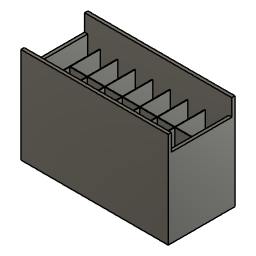
Box of WiFi (Autodesk Fusion 360 design; units mm, degrees)
Autodesk Fusion 360 part; units mm, degrees
sketch "Sketch1" plane through (0, 0, 0) normal (0, 1, 0) x (1, 0, 0)
  line L0 (0, 0) -> (139, 0)
  line L1 (139, 0) -> (139, -63)
  line L2 (139, -63) -> (0, -63)
  line L3 (0, -63) -> (0, 0)
  line L4 (0, 0) -> (139, 0)
  line L5 (139, 0) -> (139, -3)
  line L6 (139, -3) -> (0, -3)
  line L7 (0, -3) -> (0, 0)
  line L8 (0, -60) -> (139, -60)
  line L9 (139, -60) -> (139, -63)
  line L10 (139, -63) -> (0, -63)
  line L11 (0, -63) -> (0, -60)
  line L12 (136, -3) -> (139, -3)
  line L13 (139, -3) -> (139, -60)
  line L14 (139, -60) -> (136, -60)
  line L15 (136, -60) -> (136, -3)
  line L16 (0, -3) -> (3, -3)
  line L17 (3, -3) -> (3, -60)
  line L18 (3, -60) -> (0, -60)
  line L19 (0, -60) -> (0, -3)
  circle A0 centre (121.9, -46) radius 3.5
  line L20 (113.4, -3) -> (113.9, -3)
  line L21 (113.9, -3) -> (113.9, -60)
  line L22 (113.9, -60) -> (113.4, -60)
  line L23 (113.4, -60) -> (113.4, -3)
  circle A1 centre (121.9, -17) radius 3.5
  circle A2 centre (121.9, -46) radius 3.5
  line L24 (113.4, -3) -> (113.9, -3)
  line L25 (113.9, -60) -> (113.4, -60)
  line L26 (113.9, -3) -> (113.9, -60)
  circle A3 centre (121.9, -17) radius 3.5
  line L27 (113.4, -60) -> (113.4, -3)
  line L28 (96.9, -60) -> (96.9, -3)
  circle A4 centre (105.4, -46) radius 3.5
  line L29 (97.4, -60) -> (96.9, -60)
  line L30 (96.9, -3) -> (97.4, -3)
  line L31 (96.9, -3) -> (97.4, -3)
  circle A5 centre (105.4, -46) radius 3.5
  line L32 (97.4, -60) -> (96.9, -60)
  circle A6 centre (105.4, -17) radius 3.5
  line L33 (97.4, -3) -> (97.4, -60)
  line L34 (96.9, -60) -> (96.9, -3)
  circle A7 centre (105.4, -17) radius 3.5
  line L35 (97.4, -3) -> (97.4, -60)
  line L36 (80.9, -60) -> (80.4, -60)
  line L37 (80.4, -3) -> (80.9, -3)
  line L38 (80.4, -60) -> (80.4, -3)
  circle A8 centre (88.9, -17) radius 3.5
  line L39 (80.9, -3) -> (80.9, -60)
  circle A9 centre (88.9, -46) radius 3.5
  circle A10 centre (88.9, -17) radius 3.5
  line L40 (80.9, -3) -> (80.9, -60)
  line L41 (80.4, -60) -> (80.4, -3)
  line L42 (80.9, -60) -> (80.4, -60)
  line L43 (80.4, -3) -> (80.9, -3)
  circle A11 centre (88.9, -46) radius 3.5
  line L44 (63.9, -60) -> (63.9, -3)
  line L45 (63.9, -60) -> (63.9, -3)
  line L46 (64.4, -3) -> (64.4, -60)
  line L47 (64.4, -3) -> (64.4, -60)
  circle A12 centre (72.4, -46) radius 3.5
  circle A13 centre (72.4, -17) radius 3.5
  line L48 (63.9, -3) -> (64.4, -3)
  line L49 (63.9, -3) -> (64.4, -3)
  line L50 (64.4, -60) -> (63.9, -60)
  circle A14 centre (72.4, -46) radius 3.5
  circle A15 centre (72.4, -17) radius 3.5
  line L51 (64.4, -60) -> (63.9, -60)
  line L52 (47.4, -60) -> (47.4, -3)
  line L53 (47.9, -3) -> (47.9, -60)
  line L54 (47.4, -60) -> (47.4, -3)
  line L55 (47.4, -3) -> (47.9, -3)
  line L56 (47.4, -3) -> (47.9, -3)
  line L57 (47.9, -3) -> (47.9, -60)
  circle A16 centre (55.9, -17) radius 3.5
  circle A17 centre (55.9, -46) radius 3.5
  line L58 (47.9, -60) -> (47.4, -60)
  circle A18 centre (55.9, -46) radius 3.5
  circle A19 centre (55.9, -17) radius 3.5
  line L59 (47.9, -60) -> (47.4, -60)
  circle A20 centre (39.4, -17) radius 3.5
  line L60 (30.9, -3) -> (31.4, -3)
  circle A21 centre (39.4, -46) radius 3.5
  line L61 (30.9, -60) -> (30.9, -3)
  line L62 (30.9, -60) -> (30.9, -3)
  line L63 (31.4, -3) -> (31.4, -60)
  line L64 (30.9, -3) -> (31.4, -3)
  line L65 (31.4, -3) -> (31.4, -60)
  line L66 (31.4, -60) -> (30.9, -60)
  circle A22 centre (39.4, -17) radius 3.5
  circle A23 centre (39.4, -46) radius 3.5
  line L67 (31.4, -60) -> (30.9, -60)
  line L68 (14.9, -3) -> (14.9, -60)
  line L69 (14.4, -3) -> (14.9, -3)
  line L70 (14.4, -60) -> (14.4, -3)
  line L71 (14.9, -60) -> (14.4, -60)
  line L72 (14.9, -3) -> (14.9, -60)
  circle A24 centre (22.9, -46) radius 3.5
  line L73 (14.4, -60) -> (14.4, -3)
  circle A25 centre (22.9, -46) radius 3.5
  line L74 (14.4, -3) -> (14.9, -3)
  line L75 (14.9, -60) -> (14.4, -60)
  circle A26 centre (22.9, -17) radius 3.5
  circle A27 centre (22.9, -17) radius 3.5
  line L76 (130.4, -60) -> (129.9, -60)
  line L77 (129.9, -3) -> (130.4, -3)
  line L78 (130.4, -60) -> (129.9, -60)
  line L79 (129.9, -3) -> (130.4, -3)
  line L80 (129.9, -60) -> (129.9, -3)
  line L81 (130.4, -3) -> (130.4, -60)
  line L82 (129.9, -60) -> (129.9, -3)
  line L83 (130.4, -3) -> (130.4, -60)
  line L84 (14.9, -31.25) -> (129.9, -31.25)
  line L85 (129.9, -31.25) -> (129.9, -31.75)
  line L86 (129.9, -31.75) -> (14.9, -31.75)
  line L87 (14.9, -31.75) -> (14.9, -31.25)
  line L88 (120, -59) -> (124, -59)
  line L89 (124, -59) -> (124, -60)
  line L90 (124, -60) -> (120, -60)
  line L91 (120, -60) -> (120, -59)
  line L92 (103, -60) -> (107, -60)
  line L93 (107, -60) -> (107, -59)
  line L94 (107, -59) -> (103, -59)
  line L95 (103, -59) -> (103, -60)
  line L96 (21, -3) -> (25, -3)
  line L97 (25, -3) -> (25, -4)
  line L98 (25, -4) -> (21, -4)
  line L99 (21, -4) -> (21, -3)
  line L100 (37, -3) -> (41, -3)
  line L101 (41, -3) -> (41, -4)
  line L102 (41, -4) -> (37, -4)
  line L103 (37, -4) -> (37, -3)
  line L104 (21, -60) -> (25, -60)
  line L105 (25, -60) -> (25, -59)
  line L106 (25, -59) -> (21, -59)
  line L107 (21, -59) -> (21, -60)
  line L108 (37, -60) -> (41, -60)
  line L109 (41, -60) -> (41, -59)
  line L110 (41, -59) -> (37, -59)
  line L111 (37, -59) -> (37, -60)
  line L112 (103, -3) -> (107, -3)
  line L113 (107, -3) -> (107, -4)
  line L114 (107, -4) -> (103, -4)
  line L115 (103, -4) -> (103, -3)
  line L116 (120, -3) -> (124, -3)
  line L117 (124, -3) -> (124, -4)
  line L118 (124, -4) -> (120, -4)
  line L119 (120, -4) -> (120, -3)
  dimension "d1" = 139
  dimension "d2" = 63
  dimension "d3" = 139
  dimension "d4" = 3
  dimension "d5" = 139
  dimension "d6" = 3
  dimension "d7" = 7
  dimension "d8" = 14.1
  dimension "d9" = 14
  dimension "d10" = 0.5
  dimension "d11" = 8
  dimension "d12" = 7
  dimension "d13" = 14
  dimension "d14" = 7
  dimension "d15" = 0.5
  dimension "d16" = 8
  dimension "d17" = 7
  dimension "d18" = 7
  dimension "d19" = 0.5
  dimension "d20" = 8
  dimension "d21" = 7
  dimension "d22" = 7
  dimension "d23" = 0.5
  dimension "d24" = 8
  dimension "d25" = 7
  dimension "d26" = 7
  dimension "d27" = 0.5
  dimension "d28" = 8
  dimension "d29" = 7
  dimension "d30" = 7
  dimension "d31" = 0.5
  dimension "d32" = 8
  dimension "d33" = 7
  dimension "d34" = 7
  dimension "d35" = 0.5
  dimension "d36" = 8
  dimension "d37" = 7
  dimension "d38" = 7
  dimension "d39" = 0.5
  dimension "d40" = 8
  dimension "d41" = 7
  dimension "d42" = 7
  dimension "d43" = 0.5
  dimension "d44" = 8
  dimension "d45" = 7
  dimension "d46" = 7
  dimension "d47" = 0.5
  dimension "d48" = 8
  dimension "d49" = 7
  dimension "d50" = 7
  dimension "d51" = 0.5
  dimension "d52" = 8
  dimension "d53" = 7
  dimension "d54" = 7
  dimension "d55" = 0.5
  dimension "d56" = 8
  dimension "d57" = 7
  dimension "d58" = 7
  dimension "d59" = 0.5
  dimension "d60" = 8
  dimension "d61" = 7
  dimension "d62" = 7
  dimension "d63" = 0.5
  dimension "d64" = 8
  dimension "d65" = 7
  dimension "d66" = 0.5
  dimension "d67" = 0.5
  dimension "d68" = 0.5
  dimension "d69" = 31.25
  dimension "d70" = 4
  dimension "d71" = 1
  dimension "d72" = 5.9
  dimension "d73" = 4
  dimension "d74" = 1
  constraint horizontal L0
  constraint vertical L1
  constraint horizontal L2
  constraint vertical L3
  constraint coincident L0.start L3.end
  constraint horizontal L4
  constraint vertical L5
  constraint horizontal L6
  constraint vertical L7
  constraint horizontal L8
  constraint vertical L9
  constraint horizontal L10
  constraint vertical L11
  constraint horizontal L12
  constraint vertical L13
  constraint horizontal L14
  constraint vertical L15
  constraint coincident L6 L12.start
  constraint horizontal L16
  constraint vertical L17
  constraint horizontal L18
  constraint vertical L19
  constraint horizontal L20
  constraint vertical L21
  constraint horizontal L22
  constraint vertical L23
  constraint coincident L6 L20.start
  constraint horizontal L24
  constraint vertical L26
  constraint horizontal L25
  constraint vertical L27
  constraint horizontal L30
  constraint vertical L33
  constraint horizontal L29
  constraint vertical L28
  constraint horizontal L31
  constraint vertical L35
  constraint horizontal L32
  constraint vertical L34
  constraint horizontal L43
  constraint vertical L40
  constraint horizontal L42
  constraint vertical L38
  constraint horizontal L37
  constraint vertical L39
  constraint horizontal L36
  constraint vertical L41
  constraint horizontal L49
  constraint vertical L47
  constraint horizontal L50
  constraint vertical L44
  constraint horizontal L48
  constraint vertical L46
  constraint horizontal L51
  constraint vertical L45
  constraint horizontal L55
  constraint vertical L53
  constraint horizontal L58
  constraint vertical L52
  constraint horizontal L56
  constraint vertical L57
  constraint horizontal L59
  constraint vertical L54
  constraint horizontal L60
  constraint vertical L63
  constraint horizontal L66
  constraint vertical L62
  constraint horizontal L64
  constraint vertical L65
  constraint horizontal L67
  constraint vertical L61
  constraint horizontal L74
  constraint vertical L72
  constraint horizontal L75
  constraint vertical L73
  constraint horizontal L69
  constraint vertical L68
  constraint horizontal L71
  constraint vertical L70
  constraint horizontal L79
  constraint vertical L81
  constraint horizontal L78
  constraint vertical L80
  constraint horizontal L77
  constraint vertical L83
  constraint horizontal L76
  constraint vertical L82
  constraint horizontal L84
  constraint vertical L85
  constraint horizontal L86
  constraint vertical L87
  constraint coincident L82 L85.end
  constraint coincident L68 L84.start
  constraint horizontal L88
  constraint vertical L89
  constraint horizontal L90
  constraint vertical L91
  constraint coincident L8 L89.end
  constraint horizontal L92
  constraint vertical L93
  constraint horizontal L94
  constraint vertical L95
  constraint coincident L8 L92.start
  constraint horizontal L96
  constraint vertical L97
  constraint horizontal L98
  constraint vertical L99
  constraint coincident L6 L96.start
  constraint horizontal L100
  constraint vertical L101
  constraint horizontal L102
  constraint vertical L103
  constraint coincident L6 L100.start
  constraint horizontal L104
  constraint vertical L105
  constraint horizontal L106
  constraint vertical L107
  constraint coincident L8 L104.start
  constraint horizontal L108
  constraint vertical L109
  constraint horizontal L110
  constraint vertical L111
  constraint coincident L8 L108.start
  constraint horizontal L112
  constraint vertical L113
  constraint horizontal L114
  constraint vertical L115
  constraint coincident L6 L112.start
  constraint horizontal L116
  constraint vertical L117
  constraint horizontal L118
  constraint vertical L119
  constraint coincident L6 L116.start
  measures "d1" distance of L0.start L0.end
  measures "d2" distance of L0.start L2.end
  measures "d3" distance of L0.start L0.end
  measures "d4" distance of L0.start L6.end
  measures "d5" distance of L8.start L8.end
  measures "d6" distance of L8.start L2.end
  measures "d7" diameter of A0
  measures "d8" distance of L15 A0.centre
  measures "d9" distance of L8 A0.centre
  measures "d10" distance of L20.start L20.end
  measures "d11" distance of A0.centre L21
  measures "d12" diameter of A1
  measures "d13" distance of L6 A1.centre
  measures "d14" diameter of A2
  measures "d15" distance of L20.end L20.start
  measures "d16" distance of A0.centre L26
  measures "d17" diameter of A3
  measures "d18" diameter of A4
  measures "d19" distance of L30.end L28.end
  measures "d20" distance of A4.centre L33
  measures "d21" diameter of A6
  measures "d22" diameter of A5
  measures "d23" distance of L28.end L30.end
  measures "d24" distance of A4.centre L35
  measures "d25" diameter of A7
  measures "d26" diameter of A11
  measures "d27" distance of L37.end L37.start
  measures "d28" distance of A9.centre L40
  measures "d29" diameter of A10
  measures "d30" diameter of A9
  measures "d31" distance of L37.end L37.start
  measures "d32" distance of A9.centre L39
  measures "d33" diameter of A8
  measures "d34" diameter of A14
  measures "d35" distance of L46.start L44.end
  measures "d36" distance of A12.centre L47
  measures "d37" diameter of A13
  measures "d38" diameter of A12
  measures "d39" distance of L46.start L44.end
  measures "d40" distance of A12.centre L46
  measures "d41" diameter of A15
  measures "d42" diameter of A17
  measures "d43" distance of L53.start L52.end
  measures "d44" distance of A17.centre L53
  measures "d45" diameter of A19
  measures "d46" diameter of A18
  measures "d47" distance of L52.end L53.start
  measures "d48" distance of A17.centre L57
  measures "d49" diameter of A16
  measures "d50" diameter of A21
  measures "d51" distance of L60.start L60.end
  measures "d52" distance of A21.centre L63
  measures "d53" diameter of A20
  measures "d54" diameter of A23
  measures "d55" distance of L60.start L60.end
  measures "d56" distance of A21.centre L65
  measures "d57" diameter of A22
  measures "d58" diameter of A25
  measures "d59" distance of L68.start L69.start
  measures "d60" distance of A24.centre L72
  measures "d61" diameter of A26
  measures "d62" diameter of A24
  measures "d63" distance of L69.start L68.start
  measures "d64" distance of A24.centre L68
  measures "d65" diameter of A27
  measures "d66" distance of L77.end L77.start
  measures "d67" distance of L77.start L77.end
  measures "d68" distance of L84 L86
  measures "d69" distance of L4 L84
  measures "d70" distance of L89 L91
  measures "d71" distance of L8 L88
  measures "d72" distance of L82 L89
  measures "d73" distance of L117 L119
  measures "d74" distance of L6 L118
extrude "Extrude1" add sketch "Sketch1" against normal blind 3 contours L0 L1 L3 L4 L5 L6 L7 L12 L16 L20 L24 L30 L31 L37 L43 L48 L49 L55 L56 L60 L64 L69 L74 L77 L79 L96 L100 L112 L116 | L3 L6 L8 L16 L17 L18 L19 | L1 L6 L8 L12 L13 L14 L15 | L1 L2 L3 L8 L9 L10 L11 L14 L18 L22 L25 L29 L32 L36 L42 L50 L51 L58 L59 L66 L67 L71 L75 L76 L78 L90 L92 L104 L108 | L6 L8 L17 L70 L73 | L6 L8 L15 L81 L83 | L6 L8 L68 L69 L70 L71 L72 L73 L74 L75 L87 | L6 L8 L76 L77 L78 L79 L80 L81 L82 L83 L85 | L6 L61 L62 L68 L72 L84 L97 L98 L99 | L6 L21 L26 L80 L82 L84 L117 L118 L119 | L8 L61 L62 L68 L72 L86 L105 L106 L107 | L6 L96 L97 L98 L99 | L61 L62 L68 L72 L84 L86 L87 | L8 L21 L26 L80 L82 L86 L88 L89 L91 | L6 L116 L117 L118 L119 | L21 L26 L80 L82 L84 L85 L86 | L8 L104 L105 L106 L107 | L61 L62 L63 L65 L84 L86 | L6 L60 L61 L62 L63 L64 L65 L84 | L8 L88 L89 L90 L91 | L6 L20 L21 L23 L24 L26 L27 L84 | L21 L23 L26 L27 L84 L86 | L8 L61 L62 L63 L65 L66 L67 L86 | L52 L54 L63 L65 L84 L86 | L6 L52 L54 L63 L65 L84 L101 L102 L103 | L8 L21 L22 L23 L25 L26 L27 L86 | L6 L23 L27 L33 L35 L84 L113 L114 L115 | L23 L27 L33 L35 L84 L86 | L8 L52 L54 L63 L65 L86 L109 L110 L111 | L52 L53 L54 L57 L84 L86 | L6 L52 L53 L54 L55 L56 L57 L84 | L8 L23 L27 L33 L35 L86 L93 L94 L95 | L6 L28 L30 L31 L33 L34 L35 L84 | L28 L33 L34 L35 L84 L86 | L8 L52 L53 L54 L57 L58 L59 L86 | L6 L100 L101 L102 L103 | L44 L45 L53 L57 L84 L86 | L6 L44 L45 L53 L57 L84 | L8 L28 L29 L32 L33 L34 L35 L86 | L6 L112 L113 L114 L115 | L6 L28 L34 L39 L40 L84 | L28 L34 L39 L40 L84 L86 | L8 L108 L109 L110 L111 | L8 L44 L45 L53 L57 L86 | L44 L45 L46 L47 L84 L86 | L6 L44 L45 L46 L47 L48 L49 L84 | L8 L92 L93 L94 L95 | L8 L28 L34 L39 L40 L86 | L6 L37 L38 L39 L40 L41 L43 L84 | L38 L39 L40 L41 L84 L86 | L8 L44 L45 L46 L47 L50 L51 L86 | L38 L41 L46 L47 L84 L86 | L6 L38 L41 L46 L47 L84 | L8 L36 L38 L39 L40 L41 L42 L86 | L8 L38 L41 L46 L47 L86 | A0 A2 | A1 A3 | A4 A5 | A6 A7 | A8 A10 | A9 A11 | A12 A14 | A13 A15 | A16 A19 | A17 A18 | A20 A22 | A21 A23 | A24 A25 | A26 A27 makes body 1
extrude "Extrude2" add sketch "Sketch1" along normal blind 87.4 contours L0 L1 L3 L4 L5 L6 L7 L12 L16 L20 L24 L30 L31 L37 L43 L48 L49 L55 L56 L60 L64 L69 L74 L77 L79 L96 L100 L112 L116 bodies 1
extrude "Extrude3" add sketch "Sketch1" along normal blind 87.4 contours L1 L2 L3 L8 L9 L10 L11 L14 L18 L22 L25 L29 L32 L36 L42 L50 L51 L58 L59 L66 L67 L71 L75 L76 L78 L90 L92 L104 L108 bodies 1
extrude "Extrude4" add sketch "Sketch1" along normal blind 71.5 contours L1 L6 L8 L12 L13 L14 L15 bodies 1
extrude "Extrude5" add sketch "Sketch1" along normal blind 65 separate body contours L6 L8 L68 L69 L70 L71 L72 L73 L74 L75 L87 | L6 L8 L76 L77 L78 L79 L80 L81 L82 L83 L85 | L61 L62 L68 L72 L84 L86 L87 | L21 L26 L80 L82 L84 L85 L86 | L6 L60 L61 L62 L63 L64 L65 L84 | L6 L20 L21 L23 L24 L26 L27 L84 | L8 L61 L62 L63 L65 L66 L67 L86 | L52 L54 L63 L65 L84 L86 | L8 L21 L22 L23 L25 L26 L27 L86 | L23 L27 L33 L35 L84 L86 | L6 L52 L53 L54 L55 L56 L57 L84 | L6 L28 L30 L31 L33 L34 L35 L84 | L8 L52 L53 L54 L57 L58 L59 L86 | L44 L45 L53 L57 L84 L86 | L8 L28 L29 L32 L33 L34 L35 L86 | L28 L34 L39 L40 L84 L86 | L6 L44 L45 L46 L47 L48 L49 L84 | L6 L37 L38 L39 L40 L41 L43 L84 | L8 L44 L45 L46 L47 L50 L51 L86 | L38 L41 L46 L47 L84 L86 | L8 L36 L38 L39 L40 L41 L42 L86 makes body 2 at (130.4, 21.6667, 22)
extrude "Extrude6" add sketch "Sketch1" along normal blind 71.5 contours L3 L6 L8 L16 L17 L18 L19 bodies 1
extrude "Extrude7" cut sketch "Sketch1" against normal blind 15 contours A0 A2 | A1 A3 | A4 A5 | A6 A7 | A8 A10 | A9 A11 | A12 A14 | A13 A15 | A16 A19 | A17 A18 | A20 A22 | A21 A23 | A24 A25 | A26 A27 bodies 1
